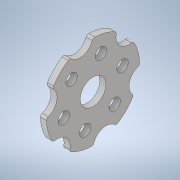
# Autodesk Inventor part: Flex_Giubo_V1
Saved by Autodesk Inventor 2021 (Build 250183000, 183)
## iProperties
Created: 2020-10-13
Part Number: Flex_Giubo_V1
Material: Generic
Document SubType Name: Modeling
Designer: PhotonUser
Density: 1 g/cm^3
Appearance: Default
Author: PhotonUser
Autodesk Inventor part; units mm, degrees
ref_plane "YZ Plane" through (0, 0, 0) normal (1, 0, 0) x (0, 1, 0)
ref_plane "XZ Plane" through (0, 0, 0) normal (0, 1, 0) x (-1, 0, 0)
ref_plane "XY Plane" through (0, 0, 0) normal (0, 0, 1) x (1, 0, 0)
sketch "Sketch1" plane through (0, 0, 0) normal (1, 0, 0) x (0, 1, 0)
  circle A0 centre (0, 0) radius 57.3659
  circle A1 centre (0, 0) radius 37.4904
  circle A2 centre (26.5097, 26.5097) radius 6.985
  line L0 (0, 0) -> (26.5097, 26.5097)
  line L1 (0, 0) -> (37.4904, 0) construction
  circle A3 centre (-9.7032, 36.2129) radius 6.985
  circle A4 centre (-36.2129, 9.7032) radius 6.985
  circle A5 centre (-26.5097, -26.5097) radius 6.985
  circle A6 centre (9.7032, -36.2129) radius 6.985
  circle A7 centre (36.2129, -9.7032) radius 6.985
  circle A8 centre (0, 0) radius 15.875
  circle A9 centre (60.1365, 16.1135) radius 15.875
  line L2 (0, 0) -> (62.2818, 0) construction
  line L3 (0, 0) -> (54.4204, 0) construction
  line L4 (0, 0) -> (47.0027, 0) construction
  line L5 (0, 0) -> (74.4134, 19.939)
  line L6 (0, 0) -> (77.0384, 0) construction
  circle A10 centre (0, 0) radius 15.875
  circle A11 centre (16.1135, 60.1365) radius 15.875
  circle A12 centre (0, 0) radius 15.875
  circle A13 centre (-44.023, 44.023) radius 15.875
  circle A14 centre (0, 0) radius 15.875
  circle A15 centre (-60.1365, -16.1135) radius 15.875
  circle A16 centre (0, 0) radius 15.875
  circle A17 centre (-16.1135, -60.1365) radius 15.875
  circle A18 centre (0, 0) radius 15.875
  circle A19 centre (44.023, -44.023) radius 15.875
  point P0 (36.2129, 9.7032)
  point P1 (49.9198, 28.264)
  point P2 (28.264, 49.9198)
  point P3 (0.4825, 57.3639)
  point P4 (-29.0998, 49.4373)
  point P5 (-49.4373, 29.0998)
  point P6 (-57.3639, -0.4825)
  point P7 (-49.9198, -28.264)
  point P8 (-28.264, -49.9198)
  point P9 (-0.4825, -57.3639)
  point P10 (29.0998, -49.4373)
  point P11 (49.4373, -29.0998)
  point P12 (57.3639, 0.4825)
  dimension "d0" = 114.7318
  dimension "d1" = 74.9808
  dimension "d2" = 13.97
  dimension "d3" = 45
  dimension "d6" = 360
  dimension "d8" = 31.75
  dimension "d12" = 31.75
  dimension "d16" = 15
  dimension "d19" = 360
  constraints: 20 centre point, 14 end point, 5 horizontal, 2 coincident, 2 equal length, 2 point on circle, 1 point on line, 38 other
  measures "d0" diameter of A0
  measures "d1" diameter of A1
  measures "d2" diameter of A2
  measures "d3" angle of L1 L0
  measures "d8" diameter of A8
  measures "d12" diameter of A9
  measures "d16" angle of L6 L5
extrude "Extrusion1" add sketch "Sketch1" along normal blind 7.5184 contours A0 A19 A17 A15 A13 A11 A9 | A1 A7 A6 A5 A4 A3 A2 L0 A8 L5 | L5 A8 L0 A2 A1
fillet "Fillet1" radius 3.175 12 edges at (3.7592, 57.3639, 0.4825) (3.7592, 49.9198, 28.264) (3.7592, 29.0998, -49.4373) (3.7592, 49.4373, -29.0998) (3.7592, -0.4825, -57.3639) (3.7592, -28.264, -49.9198) (3.7592, -49.9198, -28.264) (3.7592, -57.3639, -0.4825) (3.7592, -49.4373, 29.0998) (3.7592, -29.0998, 49.4373) (3.7592, 0.4825, 57.3639) (3.7592, 28.264, 49.9198)
body "Solid1"
